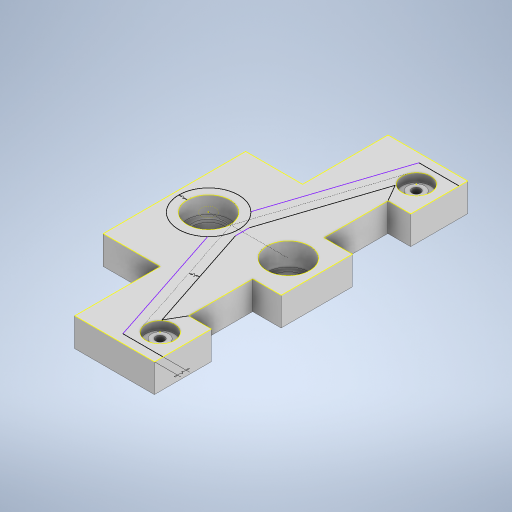
# Autodesk Inventor part: top
Saved by Autodesk Inventor 2023.1 (Build 271208000, 208)
## iProperties
Created: 2023-11-16
Part Number: top
Material: Všeobecné
Document SubType Name: Modeling
Designer: zavrel
Density: 1 g/cm^3
Appearance: Výchozí
Author: zavrel
Autodesk Inventor part; units mm, degrees
ref_plane "YZ Plane" through (0, 0, 0) normal (1, 0, 0) x (0, 1, 0)
ref_plane "XZ Plane" through (0, 0, 0) normal (0, 1, 0) x (-1, 0, 0)
ref_plane "XY Plane" through (0, 0, 0) normal (0, 0, 1) x (1, 0, 0)
sketch "Náčrt1" plane through (0, 0, 0) normal (0, 1, 0) x (-1, 0, 0)
  line L0 (-26.1298, 2.5) -> (-26.1298, 15)
  line L1 (-26.1298, 15) -> (-16.1298, 15)
  line L2 (-16.1298, 15) -> (-16.1298, 37.5)
  line L3 (-16.1298, 37.5) -> (-24.1298, 37.5)
  line L4 (-24.1298, 37.5) -> (-24.1298, 57.5)
  line L5 (-24.1298, 57.5) -> (-16.1298, 57.5)
  line L6 (-16.1298, 57.5) -> (3.8702, 57.5)
  line L7 (3.8702, 57.5) -> (3.8702, 27.5)
  line L8 (3.8702, 27.5) -> (23.8702, 27.5)
  line L9 (23.8702, 27.5) -> (23.8702, 2.5)
  line L10 (23.8702, 2.5) -> (-26.1298, 2.5) construction
  line L11 (-26.1298, 2.5) -> (-26.1298, -10)
  line L12 (-26.1298, -10) -> (-16.1298, -10)
  line L13 (-16.1298, -10) -> (-16.1298, -32.5)
  line L14 (-16.1298, -32.5) -> (-24.1298, -32.5)
  line L15 (-24.1298, -32.5) -> (-24.1298, -52.5)
  line L16 (-24.1298, -52.5) -> (-16.1298, -52.5)
  line L17 (-16.1298, -52.5) -> (3.8702, -52.5)
  line L18 (3.8702, -52.5) -> (3.8702, -22.5)
  line L19 (3.8702, -22.5) -> (23.8702, -22.5)
  line L20 (23.8702, -22.5) -> (23.8702, 2.5)
  circle A0 centre (-16.1298, 47.5) radius 5
  line L21 (-24.1298, 47.5) -> (17.4251, 47.5) construction
  circle A1 centre (-16.1298, -42.5) radius 5
  line L22 (-24.1298, -42.5) -> (17.4251, -42.5) construction
  circle A2 centre (11.8702, 2.5) radius 7.5
  circle A3 centre (-16.1298, 2.5) radius 7.5
  line L23 (-16.1298, 47.5) -> (-16.1298, -42.5) construction
  point P0 (0, 0)
  point P1 (-26.1298, 8.75)
  point P2 (-16.1298, 2.5)
  dimension "d0" = 25
  dimension "d1" = 50
  dimension "d3" = 20
  dimension "d4" = 8
  dimension "d5" = 20
  dimension "d6" = 20
  dimension "d7" = 10
  dimension "d8" = 90
  dimension "d9" = 8
  dimension "d10" = 15
  dimension "d13" = 15
  dimension "d15" = 12
  dimension "d17" = 10
  constraints: 48 end point, 12 symmetric about line, 9 perpendicular, 8 point on line, 4 centre point, 4 midpoint, 2 vertical, 1 horizontal, 1 other
  measures "d0" distance between parallel lines of L12 L1
  measures "d1" distance between parallel lines of L19 L8
  measures "d3" distance of L3.end L4.end
  measures "d4" distance between parallel lines of L13 L15
  measures "d5" distance between parallel lines of L13 L18
  measures "d6" distance between parallel lines of L18 L20
  measures "d7" diameter of A0
  measures "d8" distance of L23.end L23.start
  measures "d9" distance from line of L4 L23.start
  measures "d10" diameter of A2
  measures "d13" diameter of A3
  measures "d15" distance from line of L9 A2.centre
  measures "d17" distance of L11.end L12.end
extrude "Vysunutí1" add sketch "Náčrt1" along normal blind 10
sketch "Náčrt2" plane through (0, 0, 0) normal (0, -1, 0) x (1, 0, 0)
  line L0 (16.1298, -10) -> (16.1298, -32.5) projected
  line L1 (26.1298, -10) -> (16.1298, -10) projected
  line L2 (26.1298, 15) -> (26.1298, -10) projected
  line L3 (16.1298, 15) -> (26.1298, 15) projected
  line L4 (16.1298, 37.5) -> (16.1298, 15) projected
  line L5 (24.1298, 37.5) -> (16.1298, 37.5) projected
  line L6 (24.1298, 57.5) -> (24.1298, 37.5) projected
  line L7 (-3.8702, 57.5) -> (24.1298, 57.5) projected
  line L8 (-3.8702, 27.5) -> (-3.8702, 57.5) projected
  line L9 (-23.8702, 27.5) -> (-3.8702, 27.5) projected
  line L10 (-23.8702, -22.5) -> (-23.8702, 27.5) projected
  line L11 (-3.8702, -22.5) -> (-23.8702, -22.5) projected
  line L12 (-3.8702, -52.5) -> (-3.8702, -22.5) projected
  line L13 (24.1298, -52.5) -> (-3.8702, -52.5) projected
  line L14 (24.1298, -32.5) -> (24.1298, -52.5) projected
  line L15 (16.1298, -32.5) -> (24.1298, -32.5) projected
  circle A0 centre (16.1298, 47.5) radius 5 projected
  circle A1 centre (16.1298, -42.5) radius 5 projected
  circle A2 centre (-11.8702, 2.5) radius 7.5 projected
  circle A3 centre (16.1298, 2.5) radius 7.5 projected
  circle A4 centre (16.1298, -42.5) radius 1.5
  circle A5 centre (16.1298, 47.5) radius 5 projected
  circle A6 centre (16.1298, 47.5) radius 1.5
  point P0 (0, 0)
  dimension "d20" = 3
  constraints: 2 centre point, 2 coincident, 1 equal radius
  measures "d20" diameter of A6
extrude "Vysunutí2" add sketch "Náčrt2" against normal blind 8 contours A0 | A1
sketch "Náčrt3" plane through (0, 0, 0) normal (0, -1, 0) x (1, 0, 0)
  circle A0 centre (16.1298, 47.5) radius 1.5 projected
  circle A1 centre (16.1298, -42.5) radius 1.5 projected
  line L0 (16.1298, -10) -> (16.1298, -32.5) projected
  line L1 (26.1298, -10) -> (16.1298, -10) projected
  line L2 (26.1298, 15) -> (26.1298, -10) projected
  line L3 (16.1298, 15) -> (26.1298, 15) projected
  line L4 (16.1298, 37.5) -> (16.1298, 15) projected
  line L5 (24.1298, 37.5) -> (16.1298, 37.5) projected
  line L6 (24.1298, 57.5) -> (24.1298, 37.5) projected
  line L7 (-3.8702, 57.5) -> (24.1298, 57.5) projected
  line L8 (-3.8702, 27.5) -> (-3.8702, 57.5) projected
  line L9 (-23.8702, 27.5) -> (-3.8702, 27.5) projected
  line L10 (-23.8702, -22.5) -> (-23.8702, 27.5) projected
  line L11 (-3.8702, -22.5) -> (-23.8702, -22.5) projected
  line L12 (-3.8702, -52.5) -> (-3.8702, -22.5) projected
  line L13 (24.1298, -52.5) -> (-3.8702, -52.5) projected
  line L14 (24.1298, -32.5) -> (24.1298, -52.5) projected
  line L15 (16.1298, -32.5) -> (24.1298, -32.5) projected
  circle A2 centre (-11.8702, 2.5) radius 7.5 projected
  circle A3 centre (16.1298, 2.5) radius 7.5 projected
  circle A4 centre (16.1298, 2.5) radius 5.5
  point P0 (0, 0)
  dimension "d24" = 11
  constraints: 1 centre point, 1 coincident
  measures "d24" diameter of A4
extrude "Vysunutí3" add sketch "Náčrt3" against normal blind 2 contours A3
sketch "Náčrt4" plane through (0, 0, 0) normal (0, -1, 0) x (1, 0, 0)
  circle A0 centre (16.1298, 2.5) radius 5.5 projected
  circle A1 centre (16.1298, 47.5) radius 1.5 projected
  circle A2 centre (16.1298, -42.5) radius 1.5 projected
  line L0 (16.1298, -10) -> (16.1298, -32.5) projected
  line L1 (26.1298, -10) -> (16.1298, -10) projected
  line L2 (26.1298, 15) -> (26.1298, -10) projected
  line L3 (16.1298, 15) -> (26.1298, 15) projected
  line L4 (16.1298, 37.5) -> (16.1298, 15) projected
  line L5 (24.1298, 37.5) -> (16.1298, 37.5) projected
  line L6 (24.1298, 57.5) -> (24.1298, 37.5) projected
  line L7 (-3.8702, 57.5) -> (24.1298, 57.5) projected
  line L8 (-3.8702, 27.5) -> (-3.8702, 57.5) projected
  line L9 (-23.8702, 27.5) -> (-3.8702, 27.5) projected
  line L10 (-23.8702, -22.5) -> (-23.8702, 27.5) projected
  line L11 (-3.8702, -22.5) -> (-23.8702, -22.5) projected
  line L12 (-3.8702, -52.5) -> (-3.8702, -22.5) projected
  line L13 (24.1298, -52.5) -> (-3.8702, -52.5) projected
  line L14 (24.1298, -32.5) -> (24.1298, -52.5) projected
  line L15 (16.1298, -32.5) -> (24.1298, -32.5) projected
  circle A3 centre (-11.8702, 2.5) radius 7.5 projected
  circle A4 centre (-11.8702, 2.5) radius 2.5
  point P0 (0, 0)
  dimension "d27" = 5
  constraints: 1 centre point, 1 coincident
  measures "d27" diameter of A4
extrude "Vysunutí4" add sketch "Náčrt4" against normal blind 3 contours A3
sketch "Náčrt5" plane through (-11.8702, 3, 2.5) normal (0, 1, 0) x (1, 0, 0)
  circle A0 centre (0, 0) radius 7.5 projected
  circle A1 centre (0, 0) radius 2.5 projected
  circle A2 centre (0, 0) radius 2.5 projected
  circle A3 centre (0, 0) radius 5.5
  point P0 (11.8702, 2.5)
  dimension "d36" = 2
  constraints: 1 centre point, 1 coincident
  measures "d36" radial gap between concentric circles of A0 A3
extrude "Vysunutí5" add sketch "Náčrt5" along normal blind 1 contours A0
sketch "Náčrt6" plane through (16.1298, 8, -42.5) normal (0, 1, 0) x (1, 0, 0)
  circle A0 centre (0, -90) radius 5 projected
  circle A1 centre (0, -90) radius 1.5 projected
  circle A2 centre (0, 0) radius 5 projected
  circle A3 centre (0, 0) radius 1.5 projected
  circle A4 centre (0, -90) radius 1.5 projected
  circle A5 centre (0, -90) radius 3
  circle A6 centre (0, 0) radius 1.5 projected
  circle A7 centre (0, 0) radius 3
  point P0 (-16.1298, -42.5)
  dimension "d33" = 1.5
  constraints: 2 centre point, 2 coincident, 1 equal radius
  measures "d33" radial gap between concentric circles of A5 A1
extrude "Vysunutí6" cut sketch "Náčrt6" against normal blind 1 contours A0 | A2
sketch "Náčrt7" plane through (0, 10, 0) normal (0, 1, 0) x (1, 0, 0)
  line L0 (16.1298, 10) -> (16.1298, 32.5) projected
  line L1 (16.1298, 32.5) -> (24.1298, 32.5) projected
  line L2 (24.1298, 32.5) -> (24.1298, 52.5) projected
  line L3 (24.1298, 52.5) -> (-3.8702, 52.5) projected
  line L4 (-3.8702, 52.5) -> (-3.8702, 22.5) projected
  line L5 (-3.8702, 22.5) -> (-23.8702, 22.5) projected
  line L6 (-23.8702, 22.5) -> (-23.8702, -27.5) projected
  line L7 (-23.8702, -27.5) -> (-3.8702, -27.5) projected
  line L8 (-3.8702, -27.5) -> (-3.8702, -57.5) projected
  line L9 (-3.8702, -57.5) -> (24.1298, -57.5) projected
  line L10 (24.1298, -57.5) -> (24.1298, -37.5) projected
  line L11 (24.1298, -37.5) -> (16.1298, -37.5) projected
  line L12 (16.1298, -37.5) -> (16.1298, -15) projected
  line L13 (16.1298, -15) -> (26.1298, -15) projected
  line L14 (26.1298, -15) -> (26.1298, 10) projected
  line L15 (26.1298, 10) -> (16.1298, 10) projected
  circle A0 centre (16.1298, -47.5) radius 5 projected
  circle A1 centre (16.1298, 42.5) radius 5 projected
  circle A2 centre (-11.8702, -2.5) radius 7.5 projected
  circle A3 centre (16.1298, -2.5) radius 7.5 projected
  circle A4 centre (16.1298, -47.5) radius 5 construction
  line L16 (11.3813, -49.0657) -> (-4.7474, -0.1514) construction
  circle A5 centre (-11.8702, -2.5) radius 7.5 construction
  line L17 (-4.7474, -4.8486) -> (11.3813, 44.0657) construction
  circle A6 centre (16.1298, 42.5) radius 5 projected
  line L18 (12.6907, -43.4567) -> (0, -4.969)
  line L19 (16.1298, -37.5) -> (16.1298, -15) projected
  line L20 (16.1298, -37.5) -> (12.6907, -43.4567)
  line L21 (24.1298, 32.5) -> (24.1298, 52.5) projected
  line L22 (24.1298, -54.5) -> (10.0143, -54.5)
  circle A7 centre (-11.8702, -2.5) radius 10.5
  line L23 (10.0143, -54.5) -> (-4.6257, -10.1005)
  line L24 (0, -2.5) -> (0, -4.969)
  circle A8 centre (-11.8702, -2.5) radius 2.5 construction
  line L25 (-11.8702, -2.5) -> (16.1298, -2.5) construction
  line L26 (12.6907, 38.4567) -> (0, -0.031)
  line L27 (16.1298, 32.5) -> (12.6907, 38.4567)
  line L28 (24.1298, 49.5) -> (10.0143, 49.5)
  line L29 (10.0143, 49.5) -> (-4.6257, 5.1005)
  line L30 (0, -2.5) -> (0, -0.031)
  point P0 (0, 0)
  dimension "d39" = 3
  dimension "d43" = 3
  dimension "d44" = 3
  constraints: 26 end point, 5 symmetric about line, 3 tangent, 2 horizontal, 2 parallel, 2 point on circle, 2 point on line, 1 vertical, 9 other
  measures "d39" distance between parallel lines of L16 L18
  measures "d43" distance between parallel lines of L9 L22
